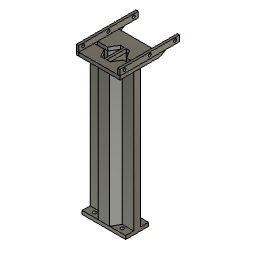
long_arm (Autodesk Fusion 360 design; units mm, degrees)
Autodesk Fusion 360 part; units mm, degrees
sketch "스케치1" plane through (0, 0, 0) normal (0, 0, 1) x (1, 0, 0)
  line L0 (0, 0) -> (38, 0)
  line L1 (38, 0) -> (38, 20)
  line L2 (38, 20) -> (0, 20)
  line L3 (0, 20) -> (0, 0)
  line L4 (0, 0) -> (0, 10)
  circle A0 centre (7, 16) radius 1.5
  circle A1 centre (31, 16) radius 1.5
  circle A2 centre (7, 4) radius 1.5
  circle A3 centre (31, 4) radius 1.5
  circle A4 centre (19, 10) radius 4
  line L5 (0, 10) -> (0, 13)
  line L6 (0, 13) -> (10, 13)
  line L7 (10, 13) -> (14.0415, 20)
  line L8 (10, 13) -> (18.0829, 13) construction
  line L9 (0, 10) -> (0, 7)
  line L10 (0, 10) -> (0, 7)
  line L11 (0, 7) -> (10, 7)
  line L12 (10, 7) -> (14.0311, 0.0179)
  line L13 (38, 10) -> (38, 13)
  line L14 (38, 13) -> (28, 13)
  line L15 (28, 13) -> (23.9585, 20)
  line L16 (28, 13) -> (36.0829, 13) construction
  line L17 (23.9585, 20) -> (14.0415, 20)
  line L18 (38, 10) -> (38, 7)
  line L19 (38, 7) -> (28, 7)
  line L20 (28, 7) -> (23.9585, 0)
  line L21 (28, 7) -> (36.0829, 7) construction
  line L22 (14.0415, 20) -> (23.9585, 20)
  line L23 (14.0311, 0.0179) -> (23.9585, 0)
  line L24 (27.134, 11.5) -> (23.0925, 18.5)
  line L25 (14.9075, 18.5) -> (23.0925, 18.5)
  line L26 (10.866, 11.5) -> (14.9075, 18.5)
  line L27 (1.5, 11.5) -> (10.866, 11.5)
  line L28 (1.5, 10) -> (1.5, 11.5)
  line L29 (1.5, 10) -> (1.5, 8.5)
  line L30 (1.5, 8.5) -> (10.866, 8.5)
  line L31 (10.866, 8.5) -> (14.8981, 1.5163)
  line L32 (14.8981, 1.5163) -> (23.0934, 1.5016)
  line L33 (27.134, 8.5) -> (23.0934, 1.5016)
  line L34 (36.5, 8.5) -> (27.134, 8.5)
  line L35 (36.5, 10) -> (36.5, 8.5)
  line L36 (36.5, 10) -> (36.5, 11.5)
  line L37 (36.5, 11.5) -> (27.134, 11.5)
  line L38 (19, 18.5) -> (20, 18.5)
  line L39 (19, 18.5) -> (18, 18.5)
  line L40 (18, 18.5) -> (17.9694, 1.5108)
  line L41 (20, 18.5) -> (19.9694, 1.5072)
  dimension "d1" = 38
  dimension "d2" = 20
  dimension "d7" = 3
  dimension "d8" = 3
  dimension "d9" = 3
  dimension "d10" = 3
  dimension "d11" = 8
  dimension "d12" = 3
  dimension "d13" = 10
  dimension "d14" = 60
  dimension "d15" = 120
  dimension "d16" = 10
  dimension "d17" = 120
  dimension "d19" = 10
  dimension "d20" = 120
  dimension "d21" = 1.5
  dimension "d22" = 1
  dimension "d23" = 1
  constraint horizontal L0
  constraint vertical L1
  constraint horizontal L2
  constraint vertical L3
  constraint coincident L0.start L3.end
  constraint midpoint L3 L4.end
  constraint midpoint L1 L13.start
  constraint horizontal L6
  constraint horizontal L8
  constraint coincident L2 L7.end
  constraint coincident L4 L9.end
  constraint coincident L1 L13.end
  constraint perpendicular L1 L14
  constraint horizontal L16
  constraint coincident L2 L15.end
  constraint horizontal L19
  constraint horizontal L21
  constraint coincident L0 L20.end
  constraint midpoint L25 L38.start
  constraint horizontal L39
  constraint coincident L32 L40.end
  constraint perpendicular L32 L40
  constraint coincident L32 L41.end
  constraint perpendicular L32 L41
  measures "d1" distance of L0.start L0.end
  measures "d2" distance of L0.start L2.end
  measures "d7" diameter of A0
  measures "d8" diameter of A1
  measures "d9" diameter of A2
  measures "d10" diameter of A3
  measures "d11" diameter of A4
  measures "d12" distance of L4.end L5.end
  measures "d13" distance of L5.end L6.end
  measures "d14" angle of L7 L8
  measures "d15" angle of L11 L12
  measures "d16" distance of L13.end L14.end
  measures "d17" angle of L15 L16
  measures "d19" distance of L18.end L19.end
  measures "d20" angle of L20 L21
  measures "d22" distance of L38.start L38.end
  measures "d23" distance of L38.start L39.end
extrude "돌출1" add sketch "스케치1" along normal blind 3 contours L0 L3 L4 L11 L12 L23 | L0 L1 L19 L20 | L1 L2 L3 L4 L5 L6 L7 L9 L10 L11 L12 L13 L14 L15 L17 L18 L19 L20 L22 L23 | L2 L3 L6 L7 | L1 L2 L14 L15 | A0 | A1 | A2 | A3 | A4 L41 | A4 L24 L25 L32 L33 L34 L35 L36 L37 L41 | A4 L40 L41 | A4 L25 L38 L39 L40 L41 | A4 L32 L40 L41 | A4 L40 | A4 L25 L26 L27 L28 L29 L30 L31 L32 L40 makes body 1
extrude "돌출2" add sketch "스케치1" against normal blind 2.5 contours A4 L41 | A4 L40 L41 | A4 L40 bodies 1
extrude "돌출3" cut sketch "스케치1" along normal blind 3 contours A0 | A1 | A2 | A3 bodies 1
extrude "돌출4" add sketch "스케치1" along normal blind 123 contours L1 L2 L3 L4 L5 L6 L7 L9 L10 L11 L12 L13 L14 L15 L17 L18 L19 L20 L22 L23 | A4 L40 L41 | A4 L25 L38 L39 L40 L41 | A4 L32 L40 L41 bodies 1
sketch "스케치2" plane through (0, 0, 123) normal (0, 0, 1) x (-1, 0, 0)
  line L0 (-36.5, -11.5) -> (-36.5, -8.5)
  line L1 (-36.5, -8.5) -> (-27.134, -8.5)
  line L2 (-27.134, -8.5) -> (-23.0934, -1.5016)
  line L3 (-23.0934, -1.5016) -> (-19.9694, -1.5072)
  line L4 (-19.9694, -1.5072) -> (-20, -18.5)
  line L5 (-20, -18.5) -> (-23.0925, -18.5)
  line L6 (-23.0925, -18.5) -> (-27.134, -11.5)
  line L7 (-27.134, -11.5) -> (-36.5, -11.5)
  line L8 (-1.5, -8.5) -> (-1.5, -11.5)
  line L9 (-1.5, -11.5) -> (-10.866, -11.5)
  line L10 (-10.866, -11.5) -> (-14.9075, -18.5)
  line L11 (-14.9075, -18.5) -> (-18, -18.5)
  line L12 (-18, -18.5) -> (-17.9694, -1.5108)
  line L13 (-17.9694, -1.5108) -> (-14.8981, -1.5163)
  line L14 (-14.8981, -1.5163) -> (-10.866, -8.5)
  line L15 (-10.866, -8.5) -> (-1.5, -8.5)
  line L16 (0, -13) -> (0, -7)
  line L17 (0, -7) -> (-10, -7)
  line L18 (-10, -7) -> (-14.0311, -0.0179)
  line L19 (-14.0311, -0.0179) -> (-23.9585, 0)
  line L20 (-23.9585, 0) -> (-28, -7)
  line L21 (-28, -7) -> (-38, -7)
  line L22 (-38, -7) -> (-38, -13)
  line L23 (-38, -13) -> (-28, -13)
  line L24 (-28, -13) -> (-23.9585, -20)
  line L25 (-23.9585, -20) -> (-14.0415, -20)
  line L26 (-14.0415, -20) -> (-10, -13)
  line L27 (-10, -13) -> (0, -13)
  line L28 (-18.9948, -0.0089) -> (-1.9949, -0.0396)
  line L29 (-1.9949, -0.0396) -> (-1.9859, 4.9604)
  line L30 (-1.9859, 4.9604) -> (-35.9859, 4.9604)
  line L31 (-35.9859, 4.9604) -> (-35.9859, -56.0396)
  line L32 (-35.9859, -56.0396) -> (-1.9859, -56.0396)
  line L33 (-1.9859, -56.0396) -> (-1.9859, 4.9604)
  line L34 (-35.9859, 4.9604) -> (-37.9859, 4.9604)
  line L35 (-1.9859, 4.9604) -> (0.0141, 4.9604)
  line L36 (0.0141, 4.9604) -> (0.0141, -56.0396)
  line L37 (0.0141, -56.0396) -> (-1.9859, -56.0396)
  line L38 (-1.9859, -56.0396) -> (-1.9859, 4.9604)
  line L39 (-37.9859, 4.9604) -> (-35.9859, 4.9604)
  line L40 (-35.9859, 4.9604) -> (-35.9859, -56.0396)
  line L41 (-35.9859, -56.0396) -> (-37.9859, -56.0396)
  line L42 (-37.9859, -56.0396) -> (-37.9859, 4.9604)
  line L43 (-1.9949, -0.0396) -> (-2.0309, -20.0395)
  line L44 (-2.0309, -20.0395) -> (-2.0309, -30.0395)
  line L45 (-2.0309, -30.0395) -> (-36.0309, -30.0395)
  line L46 (-35.9859, -56.0396) -> (-35.9859, -47.0396)
  line L47 (-35.9859, -47.0396) -> (-37.9859, -47.0396)
  line L48 (-35.9859, -47.0396) -> (0.0141, -47.0396)
  line L49 (-36.0309, -30.0395) -> (-38.0309, -30.0395)
  line L50 (-2.0309, -30.0395) -> (-0.0309, -30.0395)
  dimension "d32" = 17
  dimension "d33" = 5
  dimension "d34" = 34
  dimension "d35" = 61
  dimension "d36" = 2
  dimension "d37" = 2
  dimension "d38" = 61
  dimension "d39" = 20
  dimension "d40" = 10
  dimension "d41" = 34
  dimension "d56" = 9
  dimension "d57" = 36
  dimension "d60" = 2
  dimension "d61" = 2
  constraint midpoint L19 L28.start
  constraint parallel L19 L28
  constraint perpendicular L28 L29
  constraint horizontal L30
  constraint vertical L31
  constraint horizontal L32
  constraint vertical L33
  constraint perpendicular L31 L34
  constraint horizontal L35
  constraint vertical L36
  constraint horizontal L37
  constraint vertical L38
  constraint horizontal L39
  constraint vertical L40
  constraint horizontal L41
  constraint vertical L42
  constraint perpendicular L28 L43
  constraint perpendicular L37 L44
  constraint perpendicular L40 L45
  constraint perpendicular L41 L46
  constraint coincident L42 L47.end
  constraint perpendicular L42 L47
  constraint perpendicular L36 L48
  constraint perpendicular L42 L49
  constraint perpendicular L36 L50
  measures "d32" distance of L28.start L28.end
  measures "d33" distance of L28.end L29.end
  measures "d34" distance of L29.end L30.end
  measures "d35" distance of L29.end L32.end
  measures "d36" distance of L30.end L34.end
  measures "d37" distance of L29.end L35.end
  measures "d38" distance of L29.end L32.end
  measures "d39" distance of L28.end L43.end
  measures "d40" distance of L43.end L44.end
  measures "d41" distance of L44.end L45.end
  measures "d56" distance of L31.end L46.end
  measures "d57" distance of L46.end L48.end
  measures "d60" distance of L45.end L49.end
  measures "d61" distance of L44.end L50.end
extrude "돌출5" add sketch "스케치2" along normal blind 3 separate body contours L0 L1 L7 L21 L23 L31 L40 L42 | L0 L1 L7 L31 L40 | L1 L2 L3 L4 L5 L6 L7 L31 L40 | L1 L2 L3 L4 L5 L6 L7 L9 L10 L11 L12 L13 L14 L15 L17 L18 L19 L20 L21 L23 L24 L25 L26 L27 L28 L31 L40 L43 | L23 L31 L40 L42 L45 L49 | L23 L24 L25 L26 L27 L31 L40 L43 L44 L45 | L19 L20 L21 L28 L29 L30 L31 L40 | L21 L31 L34 L39 L40 L42 | L31 L33 L38 L40 L45 L48 L50 | L31 L40 L42 L45 L47 L49 | L31 L32 L33 L38 L40 L46 L48 | L31 L40 L41 L42 L46 L47 | L27 L33 L38 L43 L44 L50 | L16 L17 L27 L33 L35 L36 L38 L48 | L33 L36 L37 L38 L48 | L17 L18 L28 L43 | L8 L9 L15 L16 L17 L27 L33 L38 | L8 L9 L15 L33 L38 | L9 L10 L11 L12 L13 L14 L15 L43 makes body 2
extrude "돌출6" cut sketch "스케치2" along normal blind 3 contours L31 L33 L38 L40 L45 L48 L50 | L31 L32 L33 L38 L40 L46 L48 | L27 L33 L38 L43 L44 L50 bodies 2
sketch "스케치3" plane through (37.9859, 0, 0) normal (1, 0, 0) x (0, 1, 0)
  line L0 (-4.9604, 123) -> (56.0396, 123)
  line L1 (56.0396, 123) -> (56.0396, 126)
  line L2 (56.0396, 126) -> (-4.9604, 126)
  line L3 (-4.9604, 126) -> (-4.9604, 123)
  line L4 (-4.9604, 126) -> (-4.9604, 131)
  line L5 (-4.9604, 126) -> (-4.9604, 128.8)
  line L6 (-4.9604, 131) -> (56.0396, 131)
  line L7 (56.0396, 131) -> (56.0396, 126)
  line L8 (56.0396, 126) -> (-4.9604, 126)
  line L9 (-4.9604, 126) -> (-4.9604, 131)
  line L10 (-4.9604, 128.8) -> (56.0396, 128.8)
  line L11 (-4.9604, 128.8) -> (-0.9604, 128.8)
  line L12 (-0.9604, 128.8) -> (21.0396, 128.8)
  line L13 (21.0396, 128.8) -> (43.0396, 128.8)
  circle A0 centre (-0.9604, 128.8) radius 1.3
  circle A1 centre (21.0396, 128.8) radius 1.3
  circle A2 centre (43.0396, 128.8) radius 1.3
  line L14 (43.0396, 128.8) -> (47.0396, 128.8)
  line L15 (47.0396, 128.8) -> (47.0396, 131)
  line L16 (47.0396, 128.8) -> (47.0396, 126)
  line L17 (-4.9604, 123) -> (30.0396, 123)
  line L18 (30.0396, 123) -> (35.2357, 126)
  line L19 (30.0396, 123) -> (36.0396, 123) construction
  dimension "d46" = 5
  dimension "d47" = 2.8
  dimension "d48" = 61
  dimension "d49" = 4
  dimension "d50" = 22
  dimension "d51" = 22
  dimension "d52" = 2.6
  dimension "d53" = 2.6
  dimension "d54" = 2.6
  dimension "d55" = 4
  dimension "d62" = 35
  dimension "d63" = 30
  constraint coincident L2.end L3.start
  constraint perpendicular L2 L4
  constraint perpendicular L2 L5
  constraint horizontal L6
  constraint vertical L7
  constraint horizontal L8
  constraint vertical L9
  constraint coincident L1.end L2.start
  constraint horizontal L10
  constraint perpendicular L5 L11
  constraint horizontal L12
  constraint horizontal L13
  constraint coincident L11.end L12.start
  constraint coincident L12.end L13.start
  constraint coincident L13.end A2.centre
  constraint parallel L10 L14
  constraint coincident L6 L15.end
  constraint perpendicular L6 L15
  constraint coincident L8 L16.end
  constraint perpendicular L8 L16
  constraint horizontal L17
  constraint coincident L0.start L3.end
  constraint horizontal L19
  constraint coincident L8 L18.end
  measures "d46" distance of L2.end L4.end
  measures "d47" distance of L2.end L5.end
  measures "d48" distance of L5.end L10.end
  measures "d49" distance of L5.end L11.end
  measures "d50" distance of L11.end L12.end
  measures "d51" distance of L12.end L13.end
  measures "d52" diameter of A0
  measures "d53" diameter of A1
  measures "d54" diameter of A2
  measures "d55" distance of L13.end L14.end
  measures "d62" distance of L0.start L17.end
  measures "d63" angle of L18 L19
extrude "돌출7" cut sketch "스케치2" along normal blind 3 contours L31 L32 L33 L38 L40 L46 L48 | L31 L40 L41 L42 L46 L47 | L33 L36 L37 L38 L48 bodies 2
extrude "돌출8" add sketch "스케치3" against normal blind 2 separate body contours L2 L4 L5 L8 L9 L10 L11 L12 L13 A0 A1 A2 L14 L16 | L4 L6 L9 L10 L11 L12 L13 A0 A1 A2 L14 L15 makes body 3
copy_body "CopyPasteBodies1" bodies 3 makes body 4
move_body "이동1" bodies 4 to x (1, 0, 0) y (0, 1, 0) z (0, 0, 1) at (-36, 0, 0)
extrude "돌출9" cut sketch "스케치3" against normal blind 38 contours L0 L1 L2 L8 L18 bodies 2
extrude "돌출10" cut sketch "스케치2" along normal blind 3 contours L1 L2 L3 L4 L5 L6 L7 L31 L40 | L9 L10 L11 L12 L13 L14 L15 L43 bodies 2
